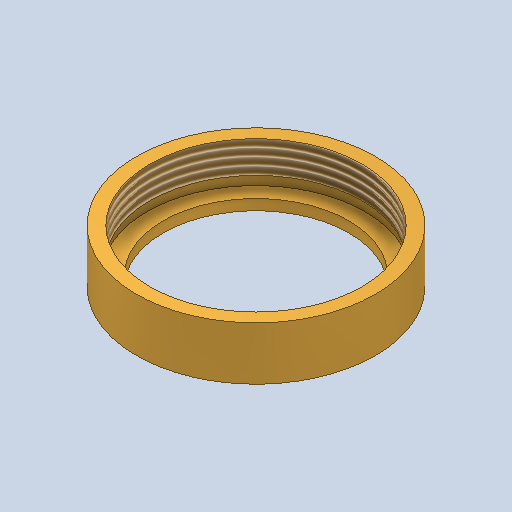
# Autodesk Inventor part: 004
Saved by Autodesk Inventor 2023 (Build 270158000, 158)
## iProperties
Created: 2022-01-03
Part Number: 004
Material: Brass, Soft Yellow
Document SubType Name: Modeling
Designer: vinicius.miguel
Density: 8.47 g/cm^3
Appearance: Brass - Satin
Author: vinicius.miguel
Autodesk Inventor part; units mm, degrees
ref_plane "YZ Plane" through (0, 0, 0) normal (1, 0, 0) x (0, 1, 0)
ref_plane "XZ Plane" through (0, 0, 0) normal (0, 1, 0) x (-1, 0, 0)
ref_plane "XY Plane" through (0, 0, 0) normal (0, 0, 1) x (1, 0, 0)
sketch "Sketch1" plane through (0, 0, 0) normal (0, 0, 1) x (1, 0, 0)
  line L0 (0, 0) -> (0, 8.5511) construction
  line L1 (17.5, 0) -> (17.5, 2)
  line L2 (17.5, 2) -> (20.5, 2)
  line L3 (20.5, 2) -> (20.5, 4)
  line L4 (20.5, 4) -> (20, 4)
  line L5 (20, 4) -> (20, 10)
  line L6 (20, 10) -> (22.5, 10)
  line L7 (22.5, 10) -> (22.5, 0)
  line L8 (22.5, 0) -> (17.5, 0)
  dimension "d0" = 35
  dimension "d1" = 2
  dimension "d2" = 2
  dimension "d3" = 40
  dimension "d4" = 0.5
  dimension "d5" = 6
  dimension "d6" = 45
  constraints: 18 end point, 7 perpendicular, 2 vertical, 1 horizontal alignment
  measures "d0" diameter of L1 L0
  measures "d1" distance of L1.start L1.end
  measures "d2" distance of L2.end L3.end
  measures "d3" diameter of L5 L0
  measures "d4" distance of L3.end L4.end
  measures "d5" distance of L4.end L5.end
  measures "d6" diameter of L7 L0
revolve "Revolution1" add sketch "Sketch1" angle 360 about axis through (0, 0, 0) along (0, 1, 0)
thread "Thread1" size "M40x1.5" class "6H" standard "ANSI Metric M Profile" length 10
body "Solid1"
